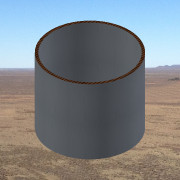
# Autodesk Inventor part: 2p3sono
Saved by Autodesk Inventor 2013 SP2 (Build 170200200, 200)
## iProperties
Company: HERA Project
Created: 2013-06-11
Part Number: 2p3sono
Material: Generic
Document SubType Name: Modeling
Designer: David DeBoer
Density: 1 g/cm^3
Description: Support stand sonotube
Mass: 2244.27 g
Surface Area: 4889.09 cm^2
Volume: 2244.27 cm^3
Author: David DeBoer
Title: Support stand sono
Autodesk Inventor part; units mm, degrees
ref_plane "YZ Plane" through (0, 0, 0) normal (1, 0, 0) x (0, 1, 0)
ref_plane "XZ Plane" through (0, 0, 0) normal (0, 1, 0) x (-1, 0, 0)
ref_plane "XY Plane" through (0, 0, 0) normal (0, 0, 1) x (1, 0, 0)
sketch "Sketch1" plane through (0, 0, 0) normal (0, 1, 0) x (-1, 0, 0)
  circle A0 centre (0, 0) radius 152.4
  circle A1 centre (0, 0) radius 142.875
  dimension "d0" = 304.8
  dimension "d2" = 9.525
  constraints: 2 centre point, 1 coincident
  measures "d0" diameter of A0
  measures "d2" radial gap between concentric circles of A1 A0
extrude "Extrusion1" add sketch "Sketch1" against normal blind 254
body "Solid1"
